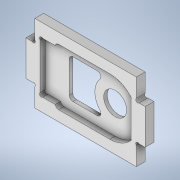
# Autodesk Inventor part: Trunk_servo_bottom_frame
Saved by Autodesk Inventor 2020.4 (Build 244396000, 396)
## iProperties
Created: 2022-01-18
Part Number: Trunk_servo_bottom_frame
Material: アセタール樹脂、黒
Document SubType Name: Modeling
Designer: Masato Kubotera
Density: 1.425 g/cm^3
Appearance: 滑らか - 淡い灰色
Mass: 11.2606 g
Surface Area: 63.2089 cm^2
Volume: 7.90215 cm^3
Author: Masato Kubotera
Autodesk Inventor part; units mm, degrees
ref_plane "YZ Plane" through (0, 0, 0) normal (1, 0, 0) x (0, 1, 0)
ref_plane "XZ Plane" through (0, 0, 0) normal (0, 1, 0) x (-1, 0, 0)
ref_plane "XY Plane" through (0, 0, 0) normal (0, 0, 1) x (1, 0, 0)
sketch "スケッチ1" plane through (0, 0, 0) normal (0, 0, 1) x (1, 0, 0)
  line L0 (12, 16) -> (-29, 16) construction
  line L1 (-31, 14) -> (-31, -14) construction
  line L2 (-29, -16) -> (12, -16) construction
  line L3 (12, -16) -> (12, 16) construction
  line L4 (12, 16) -> (-31, -16) construction
  line L5 (-31, 16) -> (12, -16) construction
  line L6 (12, 0) -> (-31, 0) construction
  circle A0 centre (0, 0) radius 10.5 construction
  arc A1 (12, 10.583) -> (0, 16) centre (0, 0) ccw construction
  line L7 (-39.5, 14.4) -> (-39.5, -14.4) construction
  arc A2 (-29, 16) -> (-31, 14) centre (-29, 14) ccw construction
  arc A3 (-31, -14) -> (-29, -16) centre (-29, -14) ccw construction
  line L8 (-39.5, 14.4) -> (-30.9596, 14.4) construction
  line L9 (-39.5, -14.4) -> (-30.9596, -14.4) construction
  line L10 (-1, 13.5) -> (-28, 13.5) construction
  line L11 (-28, 13.5) -> (-28, -13.5) construction
  line L12 (-28, -13.5) -> (-1, -13.5) construction
  line L13 (-1, -13.5) -> (-1, 13.5) construction
  line L14 (-1, 13.5) -> (-28, -13.5) construction
  line L15 (-28, 13.5) -> (-1, -13.5) construction
  circle A4 centre (-1, 13.5) radius 1.35 construction
  circle A5 centre (-28, 13.5) radius 1.35 construction
  circle A6 centre (-1, -13.5) radius 1.35 construction
  circle A7 centre (-28, -13.5) radius 1.35 construction
  arc A8 (0, -16) -> (12, -10.583) centre (0, 0) ccw construction
  arc A9 (12.05, 10.6019) -> (0, 16.05) centre (0, 0) ccw
  line L16 (12.05, 10.6019) -> (12.05, -10.6019)
  line L17 (0, 16.05) -> (-29, 16.05)
  arc A10 (-29, 16.05) -> (-31, 14.45) centre (-29, 14) ccw
  line L18 (-31, 14.45) -> (-39.55, 14.45)
  line L19 (-39.55, 14.45) -> (-39.55, -14.45)
  arc A11 (12.05, 9.8372) -> (11.5314, 11.1638) centre (11.0721, 10.2196) ccw
  arc A12 (-38.0651, 14.45) -> (-39.55, 12.9651) centre (-38.8075, 13.7075) ccw
  arc A13 (0, -16.05) -> (12.05, -10.6019) centre (0, 0) ccw
  line L20 (0, -16.05) -> (-29, -16.05)
  arc A14 (-31, -14.45) -> (-29, -16.05) centre (-29, -14) ccw
  line L21 (-31, -14.45) -> (-39.55, -14.45)
  arc A15 (11.5314, -11.1638) -> (12.05, -9.8372) centre (11.0721, -10.2196) ccw
  arc A16 (-39.55, -12.9651) -> (-38.0651, -14.45) centre (-38.8075, -13.7075) ccw
  line L22 (-42.5, 22) -> (15, 22)
  line L23 (15, 22) -> (15, -22) construction
  line L24 (15, -22) -> (-42.5, -22)
  line L25 (-42.5, -22) -> (-42.5, 22) construction
  line L26 (-42.5, 22) -> (15, -22) construction
  line L27 (15, 22) -> (-42.5, -22) construction
  line L28 (15, 10) -> (20, 10)
  line L29 (20, 10) -> (20, -10)
  line L30 (15, -10) -> (20, -10)
  arc A17 (15, 11.4849) -> (16.4849, 10) centre (15.7425, 10.7425) ccw
  arc A18 (16.4849, -10) -> (15, -11.4849) centre (15.7425, -10.7425) ccw
  line L31 (-13.75, 22) -> (-13.75, -22) construction
  line L32 (15, 11.4849) -> (15, 22)
  line L33 (15, -11.4849) -> (15, -22)
  line L34 (-42.5, 10) -> (-47.5, 10)
  line L35 (-47.5, 10) -> (-47.5, -10)
  line L36 (-42.5, -10) -> (-47.5, -10)
  arc A19 (-43.9849, 10) -> (-42.5, 11.4849) centre (-43.2425, 10.7425) ccw
  arc A20 (-42.5, -11.4849) -> (-43.9849, -10) centre (-43.2425, -10.7425) ccw
  line L37 (-42.5, 11.4849) -> (-42.5, 22)
  line L38 (-42.5, -11.4849) -> (-42.5, -22)
  circle A21 centre (0, 0) radius 6 construction
  circle A22 centre (0, 0) radius 6.5
  arc A23 (-8.5716, 7.6667) -> (-8.5716, -7.6667) centre (0, 0) ccw
  line L39 (-10.0623, 11) -> (-24, 11)
  line L40 (-26, 9) -> (-26, -9)
  line L41 (-10.0623, -11) -> (-24, -11)
  arc A24 (-24, 11) -> (-26, 9) centre (-24, 9) ccw
  arc A25 (-26, -9) -> (-24, -11) centre (-24, -9) ccw
  arc A26 (-10.0623, -11) -> (-8.5716, -7.6667) centre (-10.0623, -9) ccw
  arc A27 (-8.5716, 7.6667) -> (-10.0623, 11) centre (-10.0623, 9) ccw
  point P0 (-9.5, 0)
  point P1 (-14.5, 0)
  point P2 (12.05, 0)
  point P3 (-39.55, 0)
  point P4 (-13.75, 0)
  point P5 (12.05, -9.8372)
  point P6 (-43.9849, -10)
  point P7 (-3.3541, 11)
  point P8 (-26, 11)
  point P9 (-3.3541, -11)
  point P10 (-26, -11)
  dimension "d0" = 43
  dimension "d1" = 32
  dimension "d2" = 21
  dimension "d3" = 16
  dimension "d4" = 9.5
  dimension "d5" = 28.8
  dimension "d7" = 2
  dimension "d8" = 8.5
  dimension "d9" = 27
  dimension "d10" = 27
  dimension "d11" = 8.5
  dimension "d12" = 2.7
  dimension "d13" = 2.7
  dimension "d14" = 0.05
  dimension "d15" = 0.05
  dimension "d16" = 0.05
  dimension "d17" = 1.05
  dimension "d18" = 0.05
  dimension "d20" = 1.05
  dimension "d21" = 0.05
  dimension "d23" = 3
  dimension "d24" = 3
  dimension "d26" = 5
  dimension "d27" = 20
  dimension "d29" = 1.05
  dimension "d34" = 12
  dimension "d35" = 13
  dimension "d36" = 44
  dimension "d37" = 5
  dimension "d38" = 5
  dimension "d39" = 5
  dimension "d40" = 2
  constraints: 86 end point, 50 point on circle, 33 symmetric about line, 28 centre point, 25 point on line, 14 tangent, 12 midpoint, 9 coincident, 7 horizontal, 7 parallel, 6 perpendicular, 4 equal radius, 2 collinear, 1 vertical, 10 other
  measures "d0" distance of L2.end L4.end
  measures "d1" distance of L4.end L5.start
  measures "d2" diameter of A0
  measures "d3" radius of A1
  measures "d4" distance of point (-9.5, 0) A0.centre
  measures "d5" distance of L7.start L7.end
  measures "d7" radius of A2
  measures "d8" horizontal distance of L7.start L1.start
  measures "d9" distance of L12.end L11.end
  measures "d10" distance of L11.end L10.end
  measures "d11" horizontal distance of point (-9.5, 0) L10.start
  measures "d12" diameter of A4
  measures "d13" diameter of A5
  measures "d14" distance between parallel lines of L16 L3
  measures "d15" distance between parallel lines of L17 L0
  measures "d16" radial gap between concentric circles of A10 A2
  measures "d17" radius of A11
  measures "d18" distance between parallel lines of L18 L8
  measures "d20" radius of A12
  measures "d21" horizontal distance of L18.end L7.start
  measures "d23" horizontal distance of L0.start L22.end
  measures "d24" horizontal distance of L7.start L22.start
  measures "d26" distance of L28.start L28.end
  measures "d27" distance of L28.end L29.end
  measures "d29" radius of A17
  measures "d34" diameter of A21
  measures "d35" diameter of A22
  measures "d36" distance of L23.end L22.end
  measures "d37" radial gap between concentric circles of A23 A22
  measures "d38" distance between parallel lines of L39 L0
  measures "d39" distance between parallel lines of L40 L1
  measures "d40" radius of A24
extrude "押し出し1" add sketch "スケッチ1" along normal blind 5 contours L22 L32 A17 L28 L29 L30 A18 L33 L24 L38 A20 L36 L35 L34 A19 L37
extrude "押し出し2" add sketch "スケッチ1" along normal blind 2 contours L16 A13 L20 A14 L21 L19 L18 A10 L17 A9 | A11 L16 | A9 A11 | A15 L16 | A15 A13 | L18 A12 | L19 A12 | L19 A16 | A16 L21
equation "\"d13\" = d12"
equation "\"d15\" = d14"
equation "\"d16\" = d14"
equation "\"d18\" = d14"
equation "\"d20\" = d17"
equation "\"d21\" = d14"
equation "\"d24\" = d23"
equation "\"d29\" = d17"
equation "\"d38\" = d37"
equation "\"d39\" = d38"
